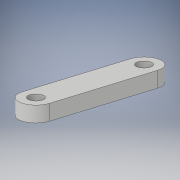
# Autodesk Inventor part: 板子6
Saved by Autodesk Inventor 2017 (Build 210142000, 142)
## iProperties
Part Number: 板子6
Material: 一般
Document SubType Name: Modeling
Designer: User
Density: 1 g/cm^3
Appearance: 預設
Author: User
Autodesk Inventor part; units mm, degrees
ref_plane "YZ Plane" through (0, 0, 0) normal (1, 0, 0) x (0, 1, 0)
ref_plane "XZ Plane" through (0, 0, 0) normal (0, 1, 0) x (-1, 0, 0)
ref_plane "XY Plane" through (0, 0, 0) normal (0, 0, 1) x (1, 0, 0)
sketch "草圖1" plane through (0, 0, 0) normal (0, 1, 0) x (-1, 0, 0)
  line L0 (0, 0) -> (0, -11)
  line L1 (0, 0) -> (0, 11)
  line L2 (0, 11) -> (0, -11) construction
  line L3 (-3.25, 11) -> (-3.25, -11)
  line L4 (3.25, -11) -> (3.25, 11)
  arc A0 (3.25, 11) -> (-3.25, 11) centre (0, 11) ccw
  arc A1 (-3.25, -11) -> (3.25, -11) centre (0, -11) ccw
  circle A2 centre (0, 11) radius 1.5
  circle A3 centre (0, -11) radius 1.5
  dimension "d7" = 11
  dimension "d8" = 11
  dimension "d9" = 3.25
  dimension "d10" = 3
  dimension "d11" = 3
  constraints: 12 end point, 4 centre point, 4 point on circle, 4 tangent, 3 vertical, 2 coincident, 1 midpoint, 1 parallel
  measures "d7" distance of L0.start L0.end
  measures "d8" distance of L0.start L1.end
  measures "d9" radius of A1
  measures "d10" diameter of A2
  measures "d11" diameter of A3
extrude "擠出1" add sketch "草圖1" along normal mid plane 3
